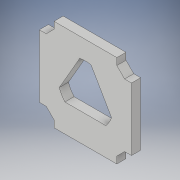
# Autodesk Inventor part: LC_objective_holder
Saved by Autodesk Inventor 2019 (Build 230136000, 136)
## iProperties
Created: 2019-10-23
Part Number: LC_objective_holder
Material: Generic
Document SubType Name: Modeling
Designer: marsikovabarbora
Density: 1 g/cm^3
Appearance: Default
Lens_diameter: 25,000 mm
Author: marsikovabarbora
Autodesk Inventor part; units mm, degrees
ref_plane "YZ Plane" through (0, 0, 0) normal (1, 0, 0) x (0, 1, 0)
ref_plane "XZ Plane" through (0, 0, 0) normal (0, 1, 0) x (-1, 0, 0)
ref_plane "XY Plane" through (0, 0, 0) normal (0, 0, 1) x (1, 0, 0)
sketch "Sketch1" plane through (0, 0, 0) normal (0, 0, 1) x (1, 0, 0)
  line L0 (-39.2988, 0) -> (59.8542, 0) construction
  line L1 (0, -36.6223) -> (0, 43.7956) construction
  line L2 (0, 0) -> (32.3074, 32.3074) construction
  line L3 (0, 0) -> (45.6895, 0) construction
  line L4 (0, 24.9041) -> (16.9, 24.9041)
  line L5 (16.9, 24.9041) -> (16.9, 21.2841)
  line L6 (16.9, 21.2841) -> (19.092, 19.092)
  line L7 (24.9041, 0) -> (24.9041, 16.9)
  line L8 (24.9041, 16.9) -> (21.2841, 16.9)
  line L9 (21.2841, 16.9) -> (19.092, 19.092)
  line L10 (0, 24.9041) -> (-16.9, 24.9041)
  line L11 (-16.9, 24.9041) -> (-16.9, 21.2841)
  line L12 (-16.9, 21.2841) -> (-19.092, 19.092)
  line L13 (-24.9041, 0) -> (-24.9041, 16.9)
  line L14 (-24.9041, 16.9) -> (-21.2841, 16.9)
  line L15 (-21.2841, 16.9) -> (-19.092, 19.092)
  line L16 (0, -24.9041) -> (16.9, -24.9041)
  line L17 (16.9, -24.9041) -> (16.9, -21.2841)
  line L18 (16.9, -21.2841) -> (19.092, -19.092)
  line L19 (24.9041, 0) -> (24.9041, -16.9)
  line L20 (24.9041, -16.9) -> (21.2841, -16.9)
  line L21 (21.2841, -16.9) -> (19.092, -19.092)
  line L22 (0, -24.9041) -> (-16.9, -24.9041)
  line L23 (-16.9, -24.9041) -> (-16.9, -21.2841)
  line L24 (-16.9, -21.2841) -> (-19.092, -19.092)
  line L25 (-24.9041, 0) -> (-24.9041, -16.9)
  line L26 (-24.9041, -16.9) -> (-21.2841, -16.9)
  line L27 (-21.2841, -16.9) -> (-19.092, -19.092)
  line L28 (17.13, 25.1341) -> (0, 25.1341)
  line L29 (0, 25.1341) -> (-17.13, 25.1341)
  line L30 (-17.13, 25.1341) -> (-17.13, 21.3793)
  line L31 (-17.13, 21.3793) -> (-19.2547, 19.2547)
  line L32 (-19.2547, 19.2547) -> (-21.3793, 17.13)
  line L33 (-21.3793, 17.13) -> (-25.1341, 17.13)
  line L34 (-25.1341, 17.13) -> (-25.1341, 0)
  line L35 (-25.1341, 0) -> (-25.1341, -17.13)
  line L36 (-25.1341, -17.13) -> (-21.3793, -17.13)
  line L37 (-21.3793, -17.13) -> (-19.2547, -19.2547)
  line L38 (-19.2547, -19.2547) -> (-17.13, -21.3793)
  line L39 (-17.13, -21.3793) -> (-17.13, -25.1341)
  line L40 (-17.13, -25.1341) -> (0, -25.1341)
  line L41 (0, -25.1341) -> (17.13, -25.1341)
  line L42 (17.13, -25.1341) -> (17.13, -21.3793)
  line L43 (17.13, -21.3793) -> (19.2547, -19.2547)
  line L44 (19.2547, -19.2547) -> (21.3793, -17.13)
  line L45 (21.3793, -17.13) -> (25.1341, -17.13)
  line L46 (25.1341, -17.13) -> (25.1341, 0)
  line L47 (25.1341, 0) -> (25.1341, 17.13)
  line L48 (25.1341, 17.13) -> (21.3793, 17.13)
  line L49 (21.3793, 17.13) -> (19.2547, 19.2547)
  line L50 (19.2547, 19.2547) -> (17.13, 21.3793)
  line L51 (17.13, 21.3793) -> (17.13, 25.1341)
  dimension "d27" = 45
  dimension "d28" = 16.9
  dimension "d29" = 3.62
  dimension "d30" = 3.1
  dimension "d31" = 0.23
  constraints: 100 end point, 20 symmetric about line, 3 perpendicular, 2 horizontal, 2 point on line, 1 equal length, 23 other
  measures "d27" angle of L3 L2
  measures "d28" distance of L4.start L4.end
  measures "d29" distance of L4.end L5.end
  measures "d30" distance of L5.end L6.end
  measures "d31" distance between parallel lines of L4 L28
extrude "Extrusion1" add sketch "Sketch1" along normal blind 5 contours L4 L5 L6 L9 L8 L7 L19 L20 L21 L18 L17 L16 L22 L23 L24 L27 L26 L25 L13 L14 L15 L12 L11 L10 | L51 L50 L49 L48 L47 L46 L45 L44 L43 L42 L41 L40 L39 L38 L37 L36 L35 L34 L33 L32 L31 L30 L29 L28
hole "Hole1" at (0, 0, 0) direction (0, 0, 1) diameter 30 end through all
sketch "Sketch2" plane through (0, 0, 0) normal (0, 0, -1) x (-1, 0, 0)
  circle A0 centre (0, 0) radius 15 projected
  line L0 (3.0701, 14.6825) -> (14.2504, -4.6825)
  line L1 (11.1803, -10) -> (-11.1803, -10)
  line L2 (-14.2504, -4.6825) -> (-3.0701, 14.6825)
  circle A1 centre (0, 0) radius 10 construction
  circle A2 centre (0, 0) radius 15 construction
  circle A3 centre (0, 0) radius 15 construction
  arc A4 (14.2504, -4.6825) -> (3.0701, 14.6825) centre (0, 0) ccw
  arc A5 (-11.1803, -10) -> (11.1803, -10) centre (0, 0) ccw
  arc A6 (-3.0701, 14.6825) -> (-14.2504, -4.6825) centre (0, 0) ccw
  dimension "d22" = 20
  constraints: 7 point on circle, 6 end point, 4 centre point, 2 coincident, 1 point on line, 1 tangent, 16 other
  measures "d22" diameter of A1
extrude "Extrusion2" add sketch "Sketch2" against normal up to surface (5 mm away) contours A0 L0 | L2 A0 | A0 L1
equation "\"Lens_diameter\" = 25"
body "Solid1"
